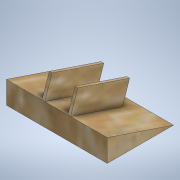
# Autodesk Inventor part: WOODEN CORRECT SLIDER
Saved by Autodesk Inventor 2021 (Build 250183000, 183)
## iProperties
Created: 2021-07-15
Part Number: WOODEN CORRECT SLIDER
Material: Generic
Document SubType Name: Modeling
Designer: HP
Density: 1 g/cm^3
Appearance: Plywood - Weathered
Author: HP
Autodesk Inventor part; units mm, degrees
ref_plane "YZ Plane" through (0, 0, 0) normal (1, 0, 0) x (0, 1, 0)
ref_plane "XZ Plane" through (0, 0, 0) normal (0, 1, 0) x (-1, 0, 0)
ref_plane "XY Plane" through (0, 0, 0) normal (0, 0, 1) x (1, 0, 0)
sketch "Sketch1" plane through (0, 0, 0) normal (1, 0, 0) x (0, 1, 0)
  line L0 (0, 20.6375) -> (25.4, 20.6375)
  line L1 (0, 20.6375) -> (0, -54.5465)
  line L2 (0, -54.5465) -> (25.4, 20.6375)
  point P0 (0, 0)
  dimension "d0" = 25.4
  dimension "d1" = 75.184
  constraints: 6 end point, 1 horizontal, 1 vertical
  measures "d0" distance of L0.start L0.end
  measures "d1" distance of L0.start L1.end
extrude "Extrusion1" add sketch "Sketch1" along normal blind 114.3
sketch "Sketch2" plane through (0, 25.4, 20.6375) normal (0, 0.9474, -0.3201) x (1, 0, 0)
  line L0 (0, 79.3586) -> (0, 0) projected
  line L1 (0, 0) -> (114.3, 0) projected
  line L2 (114.3, 79.3586) -> (114.3, 0) projected
  line L3 (0, 79.3586) -> (114.3, 79.3586) projected
  line L4 (0, 0) -> (114.3, 0) projected
  line L5 (72.8666, 0) -> (69.7688, 0)
  line L6 (69.7688, 0) -> (69.7688, 61.9125)
  line L7 (69.7688, 61.9125) -> (72.8666, 61.9125)
  line L8 (72.8666, 61.9125) -> (72.8666, 0)
  line L9 (43.6373, 0) -> (40.4623, 0)
  line L10 (40.4623, 0) -> (40.4623, 61.9125)
  line L11 (40.4623, 61.9125) -> (43.6373, 61.9125)
  line L12 (43.6373, 61.9125) -> (43.6373, 0)
  point P0 (0, 27.6815)
  dimension "d4" = 3.175
  constraints: 16 end point, 3 parallel, 2 horizontal, 2 perpendicular, 2 point on line
  measures "d4" distance of L10.end L11.end
extrude "Extrusion2" add sketch "Sketch2" along normal blind 25.4 contours L10 L11 L12 L1 | L1 L6 L7 L8
body "Solid1"
